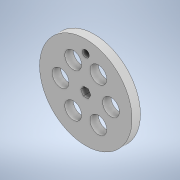
# Autodesk Inventor part: driveForPiston
Saved by Autodesk Inventor 2020.2 (Build 242310000, 310)
## iProperties
Created: 2020-01-13
Part Number: driveForPiston
Material: Generic
Document SubType Name: Modeling
Designer: robst
Density: 1 g/cm^3
Appearance: Default
Author: robst
Autodesk Inventor part; units mm, degrees
ref_plane "YZ Plane" through (0, 0, 0) normal (1, 0, 0) x (0, 1, 0)
ref_plane "XZ Plane" through (0, 0, 0) normal (0, 1, 0) x (-1, 0, 0)
ref_plane "XY Plane" through (0, 0, 0) normal (0, 0, 1) x (1, 0, 0)
sketch "Sketch1" plane through (0, 0, 0) normal (0, 0, 1) x (1, 0, 0)
  circle A0 centre (0, 0) radius 69.85
  line L0 (7.6256, 0) -> (3.8128, -6.604)
  line L1 (3.8128, -6.604) -> (-3.8128, -6.604)
  line L2 (-3.8128, -6.604) -> (-7.6256, 0)
  line L3 (-7.6256, 0) -> (-3.8128, 6.604)
  line L4 (-3.8128, 6.604) -> (3.8128, 6.604)
  line L5 (3.8128, 6.604) -> (7.6256, 0)
  circle A1 centre (0, 50.8) radius 5.2705
  dimension "d0" = 139.7
  dimension "d1" = 13.208
  dimension "d2" = 10.541
  dimension "d5" = 50.8
  constraints: 12 end point, 2 centre point, 2 coincident, 1 horizontal, 13 other
  measures "d0" diameter of A0
  measures "d1" distance between parallel lines of L1 L4
  measures "d2" diameter of A1
  measures "d5" distance of A1.centre point (0, 0)
extrude "Extrusion1" add sketch "Sketch1" along normal mid plane 12.7
sketch "Sketch2" plane through (0, 0, 6.35) normal (0, 0, 1) x (1, 0, 0)
  circle A0 centre (-38.1, 0) radius 12.7
  circle A1 centre (-19.05, -32.9956) radius 12.7
  circle A2 centre (19.05, -32.9956) radius 12.7
  circle A3 centre (38.1, 0) radius 12.7
  circle A4 centre (19.05, 32.9956) radius 12.7
  circle A5 centre (-19.05, 32.9956) radius 12.7
  point P0 (0, 0)
  dimension "d6" = 25.4
  dimension "d7" = 38.1
  dimension "d10" = 360
  constraints: 6 centre point, 13 other
  measures "d6" diameter of A0
  measures "d7" distance of A0.centre point (0, 0)
extrude "Extrusion2" cut sketch "Sketch2" against normal through all
body "Solid1"
